Autodesk Fusion 360 part; units mm, degrees
(part 11 of 18)
  line L7284 (210.9744, -11.8381) -> (210.7744, -11.8381)
  line L7285 (210.7744, -11.8381) -> (210.7744, -12.5031)
  line L7286 (211.1744, -11.8381) -> (211.1744, -12.5031)
  line L7287 (211.1744, -12.5031) -> (211.3744, -12.5031)
  line L7288 (211.3744, -12.5031) -> (211.3744, -11.8381)
  line L7289 (211.3744, -11.8381) -> (211.1744, -11.8381)
  line L7290 (208.5746, -11.8381) -> (208.3746, -11.8381)
  line L7291 (208.3746, -11.8381) -> (208.3746, -12.5031)
  line L7292 (208.5746, -12.5031) -> (208.5746, -11.8381)
  line L7293 (208.3746, -12.5031) -> (208.5746, -12.5031)
  line L7294 (213.3744, -11.8381) -> (213.1744, -11.8381)
  line L7295 (213.1744, -11.8381) -> (213.1744, -12.5031)
  line L7296 (213.3744, -12.5031) -> (213.3744, -11.8381)
  line L7297 (213.1744, -12.5031) -> (213.3744, -12.5031)
  line L7298 (210.3746, -12.5031) -> (210.5746, -12.5031)
  line L7299 (210.5746, -11.8381) -> (210.3746, -11.8381)
  line L7300 (210.5746, -12.5031) -> (210.5746, -11.8381)
  line L7301 (210.3746, -11.8381) -> (210.3746, -12.5031)
  line L7302 (212.9744, -11.8381) -> (212.7744, -11.8381)
  line L7303 (212.7744, -11.8381) -> (212.7744, -12.5031)
  line L7304 (212.7744, -12.5031) -> (212.9744, -12.5031)
  line L7305 (212.9744, -12.5031) -> (212.9744, -11.8381)
  line L7306 (210.1745, -12.5031) -> (210.1745, -11.8381)
  line L7307 (209.9745, -12.5031) -> (210.1745, -12.5031)
  line L7308 (210.1745, -11.8381) -> (209.9745, -11.8381)
  line L7309 (209.9745, -11.8381) -> (209.9745, -12.5031)
  line L7310 (212.5746, -11.8381) -> (212.3746, -11.8381)
  line L7311 (212.3746, -12.5031) -> (212.5746, -12.5031)
  line L7312 (212.3746, -11.8381) -> (212.3746, -12.5031)
  line L7313 (212.5746, -12.5031) -> (212.5746, -11.8381)
  line L7314 (209.5745, -11.8381) -> (209.5745, -12.5031)
  line L7315 (209.7745, -12.5031) -> (209.7745, -11.8381)
  line L7316 (209.5745, -12.5031) -> (209.7745, -12.5031)
  line L7317 (209.7745, -11.8381) -> (209.5745, -11.8381)
  line L7318 (211.5745, -11.8381) -> (211.5745, -12.5031)
  line L7319 (211.5745, -12.5031) -> (211.7745, -12.5031)
  line L7320 (211.7745, -11.8381) -> (211.5745, -11.8381)
  line L7321 (211.7745, -12.5031) -> (211.7745, -11.8381)
  line L7322 (208.9744, -12.5031) -> (208.9744, -11.8381)
  line L7323 (208.9744, -11.8381) -> (208.7744, -11.8381)
  line L7324 (208.7744, -11.8381) -> (208.7744, -12.5031)
  line L7325 (208.7744, -12.5031) -> (208.9744, -12.5031)
  line L7326 (211.9745, -11.8381) -> (211.9745, -12.5031)
  line L7327 (212.1745, -12.5031) -> (212.1745, -11.8381)
  line L7328 (212.1745, -11.8381) -> (211.9745, -11.8381)
  line L7329 (211.9745, -12.5031) -> (212.1745, -12.5031)
  line L7330 (209.3744, -12.5031) -> (209.3744, -11.8381)
  line L7331 (209.1744, -12.5031) -> (209.3744, -12.5031)
  line L7332 (209.1744, -11.8381) -> (209.1744, -12.5031)
  line L7333 (209.3744, -11.8381) -> (209.1744, -11.8381)
  line L7334 (209.4745, -7.1629) -> (212.6745, -7.1629)
  line L7335 (212.6745, -7.1629) -> (212.6745, -10.3629)
  line L7336 (212.6745, -10.3629) -> (209.4745, -10.3629)
  line L7337 (209.4745, -10.3629) -> (209.4745, -7.1629)
  line L7338 (188.0514, -6.559) -> (188.4214, -6.559)
  line L7339 (188.0514, -7.131) -> (188.1014, -7.181)
  line L7340 (188.4214, -6.889) -> (188.0514, -6.889)
  line L7341 (188.1014, -7.181) -> (188.9014, -7.181)
  line L7342 (188.4214, -6.559) -> (188.4214, -6.889)
  line L7343 (188.9514, -6.331) -> (188.9014, -6.281)
  line L7344 (188.9014, -7.181) -> (188.9514, -7.131)
  line L7345 (188.9014, -6.281) -> (188.1014, -6.281)
  line L7346 (188.0514, -6.889) -> (188.0514, -7.131)
  line L7347 (188.9514, -7.131) -> (188.9514, -6.331)
  line L7348 (188.1014, -6.281) -> (188.0514, -6.331)
  line L7349 (188.0514, -6.331) -> (188.0514, -6.559)
  line L7350 (187.3114, -7.181) -> (187.3614, -7.131)
  line L7351 (186.4614, -7.131) -> (186.5114, -7.181)
  line L7352 (186.5114, -6.281) -> (186.4614, -6.331)
  line L7353 (186.9914, -6.903) -> (186.9914, -6.573)
  line L7354 (186.5114, -7.181) -> (187.3114, -7.181)
  line L7355 (187.3614, -6.331) -> (187.3114, -6.281)
  line L7356 (187.3114, -6.281) -> (186.5114, -6.281)
  line L7357 (187.3614, -7.131) -> (187.3614, -6.903)
  line L7358 (186.4614, -6.331) -> (186.4614, -7.131)
  line L7359 (186.9914, -6.573) -> (187.3614, -6.573)
  line L7360 (187.3614, -6.903) -> (186.9914, -6.903)
  line L7361 (187.3614, -6.573) -> (187.3614, -6.331)
  line L7362 (181.9393, -7.181) -> (182.7393, -7.181)
  line L7363 (181.9393, -6.281) -> (181.8894, -6.331)
  line L7364 (182.4194, -6.573) -> (182.7894, -6.573)
  line L7365 (181.8894, -6.331) -> (181.8894, -7.131)
  line L7366 (182.7894, -6.331) -> (182.7393, -6.281)
  line L7367 (182.7894, -6.903) -> (182.4194, -6.903)
  line L7368 (182.7894, -7.131) -> (182.7894, -6.903)
  line L7369 (182.7393, -6.281) -> (181.9393, -6.281)
  line L7370 (182.4194, -6.903) -> (182.4194, -6.573)
  line L7371 (182.7393, -7.181) -> (182.7894, -7.131)
  line L7372 (182.7894, -6.573) -> (182.7894, -6.331)
  line L7373 (181.8894, -7.131) -> (181.9393, -7.181)
  line L7374 (183.8494, -6.559) -> (183.8494, -6.889)
  line L7375 (183.4794, -6.559) -> (183.8494, -6.559)
  line L7376 (183.4794, -6.331) -> (183.4794, -6.559)
  line L7377 (184.3294, -6.281) -> (183.5294, -6.281)
  line L7378 (183.4794, -6.889) -> (183.4794, -7.131)
  line L7379 (183.4794, -7.131) -> (183.5294, -7.181)
  line L7380 (183.5294, -7.181) -> (184.3294, -7.181)
  line L7381 (184.3294, -7.181) -> (184.3794, -7.131)
  line L7382 (183.8494, -6.889) -> (183.4794, -6.889)
  line L7383 (183.5294, -6.281) -> (183.4794, -6.331)
  line L7384 (184.3794, -6.331) -> (184.3294, -6.281)
  line L7385 (184.3794, -7.131) -> (184.3794, -6.331)
  line L7386 (-10.6934, -88.5446) -> (-10.6934, 1.6256)
  line L7387 (222.987, 1.6256) -> (222.987, -88.5446)
  line L7388 (-10.6934, 1.6256) -> (222.987, 1.6256)
  line L7389 (222.987, -88.5446) -> (-10.6934, -88.5446)
  arc A1072 (188.2393, -3.84) -> (188.8893, -3.84) centre (188.5643, -3.84) ccw
  arc A1073 (188.8893, -3.84) -> (188.2393, -3.84) centre (188.5643, -3.84) ccw
  arc A1074 (182.4592, -3.84) -> (183.1092, -3.84) centre (182.7842, -3.84) ccw
  arc A1075 (183.1092, -3.84) -> (182.4592, -3.84) centre (182.7842, -3.84) ccw
  arc A1076 (194.3974, -57.5184) -> (189.3974, -57.5184) centre (191.8974, -57.5184) ccw
  arc A1077 (189.3974, -57.5184) -> (194.3974, -57.5184) centre (191.8974, -57.5184) ccw
  arc A1078 (170.3473, -76.5812) -> (175.3474, -76.5812) centre (172.8473, -76.5812) ccw
  arc A1079 (175.3474, -76.5812) -> (170.3473, -76.5812) centre (172.8473, -76.5812) ccw
  arc A1080 (175.3474, -57.5184) -> (170.3473, -57.5184) centre (172.8473, -57.5184) ccw
  arc A1081 (170.3473, -57.5184) -> (175.3474, -57.5184) centre (172.8473, -57.5184) ccw
  arc A1082 (175.3474, -38.4557) -> (170.3473, -38.4557) centre (172.8473, -38.4557) ccw
  arc A1083 (170.3473, -38.4557) -> (175.3474, -38.4557) centre (172.8473, -38.4557) ccw
  arc A1084 (170.3473, -19.4056) -> (175.3474, -19.4056) centre (172.8473, -19.4056) ccw
  arc A1085 (175.3474, -19.4056) -> (170.3473, -19.4056) centre (172.8473, -19.4056) ccw
  arc A1086 (151.2973, -76.5812) -> (156.2973, -76.5812) centre (153.7973, -76.5812) ccw
  arc A1087 (156.2973, -76.5812) -> (151.2973, -76.5812) centre (153.7973, -76.5812) ccw
  arc A1088 (156.2973, -38.4557) -> (151.2973, -38.4557) centre (153.7973, -38.4557) ccw
  arc A1089 (151.2973, -38.4557) -> (156.2973, -38.4557) centre (153.7973, -38.4557) ccw
  arc A1090 (156.2973, -57.5184) -> (151.2973, -57.5184) centre (153.7973, -57.5184) ccw
  arc A1091 (151.2973, -57.5184) -> (156.2973, -57.5184) centre (153.7973, -57.5184) ccw
  arc A1092 (156.2973, -19.4056) -> (151.2973, -19.4056) centre (153.7973, -19.4056) ccw
  arc A1093 (151.2973, -19.4056) -> (156.2973, -19.4056) centre (153.7973, -19.4056) ccw
  arc A1094 (132.2473, -57.5184) -> (137.2473, -57.5184) centre (134.7473, -57.5184) ccw
  arc A1095 (137.2473, -57.5184) -> (132.2473, -57.5184) centre (134.7473, -57.5184) ccw
  arc A1096 (137.2473, -38.4557) -> (132.2473, -38.4557) centre (134.7473, -38.4557) ccw
  arc A1097 (132.2473, -38.4557) -> (137.2473, -38.4557) centre (134.7473, -38.4557) ccw
  arc A1098 (132.2473, -19.4056) -> (137.2473, -19.4056) centre (134.7473, -19.4056) ccw
  arc A1099 (137.2473, -19.4056) -> (132.2473, -19.4056) centre (134.7473, -19.4056) ccw
  arc A1100 (132.2473, -76.5812) -> (137.2473, -76.5812) centre (134.7473, -76.5812) ccw
  arc A1101 (137.2473, -76.5812) -> (132.2473, -76.5812) centre (134.7473, -76.5812) ccw
  arc A1102 (118.1972, -76.5812) -> (113.1972, -76.5812) centre (115.6972, -76.5812) ccw
  arc A1103 (113.1972, -76.5812) -> (118.1972, -76.5812) centre (115.6972, -76.5812) ccw
  line L7390 (118.1972, -76.5812) -> (118.1972, -76.5812)
  arc A1104 (118.1972, -57.5184) -> (113.1972, -57.5184) centre (115.6972, -57.5184) ccw
  line L7391 (118.1972, -57.5184) -> (118.1972, -57.5184)
  arc A1105 (113.1972, -57.5184) -> (118.1972, -57.5184) centre (115.6972, -57.5184) ccw
  arc A1106 (113.1972, -19.4056) -> (118.1972, -19.4056) centre (115.6972, -19.4056) ccw
  arc A1107 (118.1972, -19.4056) -> (113.1972, -19.4056) centre (115.6972, -19.4056) ccw
  line L7392 (118.1972, -19.4056) -> (118.1972, -19.4056)
  line L7393 (118.1972, -38.4557) -> (118.1972, -38.4557)
  arc A1108 (113.1972, -38.4557) -> (118.1972, -38.4557) centre (115.6972, -38.4557) ccw
  arc A1109 (118.1972, -38.4557) -> (113.1972, -38.4557) centre (115.6972, -38.4557) ccw
  arc A1110 (94.1472, -19.4056) -> (99.1472, -19.4056) centre (96.6472, -19.4056) ccw
  arc A1111 (99.1472, -19.4056) -> (94.1472, -19.4056) centre (96.6472, -19.4056) ccw
  line L7394 (99.1472, -19.4056) -> (99.1472, -19.4056)
  line L7395 (99.1472, -38.4557) -> (99.1472, -38.4557)
  arc A1112 (94.1472, -38.4557) -> (99.1472, -38.4557) centre (96.6472, -38.4557) ccw
  arc A1113 (99.1472, -38.4557) -> (94.1472, -38.4557) centre (96.6472, -38.4557) ccw
  line L7396 (99.1472, -76.5812) -> (99.1472, -76.5812)
  arc A1114 (99.1472, -76.5812) -> (94.1472, -76.5812) centre (96.6472, -76.5812) ccw
  arc A1115 (94.1472, -76.5812) -> (99.1472, -76.5812) centre (96.6472, -76.5812) ccw
  line L7397 (99.1472, -57.5184) -> (99.1472, -57.5184)
  arc A1116 (99.1472, -57.5184) -> (94.1472, -57.5184) centre (96.6472, -57.5184) ccw
  arc A1117 (94.1472, -57.5184) -> (99.1472, -57.5184) centre (96.6472, -57.5184) ccw
  arc A1118 (194.3974, -76.5812) -> (189.3974, -76.5812) centre (191.8974, -76.5812) ccw
  arc A1119 (189.3974, -76.5812) -> (194.3974, -76.5812) centre (191.8974, -76.5812) ccw
  arc A1120 (189.3974, -19.4056) -> (194.3974, -19.4056) centre (191.8974, -19.4056) ccw
  arc A1121 (194.3974, -19.4056) -> (189.3974, -19.4056) centre (191.8974, -19.4056) ccw
  line L7398 (80.0972, -76.5812) -> (80.0972, -76.5812)
  arc A1122 (75.0972, -76.5812) -> (80.0972, -76.5812) centre (77.5972, -76.5812) ccw
  arc A1123 (80.0972, -76.5812) -> (75.0972, -76.5812) centre (77.5972, -76.5812) ccw
  arc A1124 (80.0972, -38.4557) -> (75.0972, -38.4557) centre (77.5972, -38.4557) ccw
  line L7399 (80.0972, -38.4557) -> (80.0972, -38.4557)
  arc A1125 (75.0972, -38.4557) -> (80.0972, -38.4557) centre (77.5972, -38.4557) ccw
  arc A1126 (75.0972, -19.4056) -> (80.0972, -19.4056) centre (77.5972, -19.4056) ccw
  line L7400 (80.0972, -19.4056) -> (80.0972, -19.4056)
  arc A1127 (80.0972, -19.4056) -> (75.0972, -19.4056) centre (77.5972, -19.4056) ccw
  arc A1128 (80.0972, -57.5184) -> (75.0972, -57.5184) centre (77.5972, -57.5184) ccw
  arc A1129 (75.0972, -57.5184) -> (80.0972, -57.5184) centre (77.5972, -57.5184) ccw
  line L7401 (80.0972, -57.5184) -> (80.0972, -57.5184)
  arc A1130 (56.0471, -76.5812) -> (61.0471, -76.5812) centre (58.5471, -76.5812) ccw
  arc A1131 (61.0471, -76.5812) -> (56.0471, -76.5812) centre (58.5471, -76.5812) ccw
  arc A1132 (61.0471, -57.5184) -> (56.0471, -57.5184) centre (58.5471, -57.5184) ccw
  arc A1133 (56.0471, -57.5184) -> (61.0471, -57.5184) centre (58.5471, -57.5184) ccw
  arc A1134 (61.0471, -38.4557) -> (56.0471, -38.4557) centre (58.5471, -38.4557) ccw
  arc A1135 (56.0471, -38.4557) -> (61.0471, -38.4557) centre (58.5471, -38.4557) ccw
  arc A1136 (41.9971, -57.5184) -> (36.9971, -57.5184) centre (39.4971, -57.5184) ccw
  arc A1137 (36.9971, -57.5184) -> (41.9971, -57.5184) centre (39.4971, -57.5184) ccw
  arc A1138 (36.9971, -76.5812) -> (41.9971, -76.5812) centre (39.4971, -76.5812) ccw
  arc A1139 (41.9971, -76.5812) -> (36.9971, -76.5812) centre (39.4971, -76.5812) ccw
  arc A1140 (22.947, -76.5812) -> (17.947, -76.5812) centre (20.447, -76.5812) ccw
  arc A1141 (17.947, -76.5812) -> (22.947, -76.5812) centre (20.447, -76.5812) ccw
  arc A1142 (3.897, -76.5812) -> (-1.103, -76.5812) centre (1.397, -76.5812) ccw
  arc A1143 (-1.103, -76.5812) -> (3.897, -76.5812) centre (1.397, -76.5812) ccw
  arc A1144 (61.0471, -19.4056) -> (56.0471, -19.4056) centre (58.5471, -19.4056) ccw
  arc A1145 (56.0471, -19.4056) -> (61.0471, -19.4056) centre (58.5471, -19.4056) ccw
  arc A1146 (36.9971, -38.4557) -> (41.9971, -38.4557) centre (39.4971, -38.4557) ccw
  arc A1147 (41.9971, -38.4557) -> (36.9971, -38.4557) centre (39.4971, -38.4557) ccw
  arc A1148 (36.9971, -19.4056) -> (41.9971, -19.4056) centre (39.4971, -19.4056) ccw
  arc A1149 (41.9971, -19.4056) -> (36.9971, -19.4056) centre (39.4971, -19.4056) ccw
  arc A1150 (22.947, -19.4056) -> (17.947, -19.4056) centre (20.447, -19.4056) ccw
  arc A1151 (17.947, -19.4056) -> (22.947, -19.4056) centre (20.447, -19.4056) ccw
  arc A1152 (22.947, -57.5184) -> (17.947, -57.5184) centre (20.447, -57.5184) ccw
  arc A1153 (17.947, -57.5184) -> (22.947, -57.5184) centre (20.447, -57.5184) ccw
  arc A1154 (17.947, -38.4557) -> (22.947, -38.4557) centre (20.447, -38.4557) ccw
  arc A1155 (22.947, -38.4557) -> (17.947, -38.4557) centre (20.447, -38.4557) ccw
  arc A1156 (3.897, -19.4056) -> (-1.103, -19.4056) centre (1.397, -19.4056) ccw
  arc A1157 (-1.103, -19.4056) -> (3.897, -19.4056) centre (1.397, -19.4056) ccw
  arc A1158 (-1.103, -38.4557) -> (3.897, -38.4557) centre (1.397, -38.4557) ccw
  arc A1159 (3.897, -38.4557) -> (-1.103, -38.4557) centre (1.397, -38.4557) ccw
  arc A1160 (3.897, -57.5184) -> (-1.103, -57.5184) centre (1.397, -57.5184) ccw
  arc A1161 (-1.103, -57.5184) -> (3.897, -57.5184) centre (1.397, -57.5184) ccw
  arc A1162 (208.4474, -57.5184) -> (213.4474, -57.5184) centre (210.9474, -57.5184) ccw
  arc A1163 (213.4474, -57.5184) -> (208.4474, -57.5184) centre (210.9474, -57.5184) ccw
  arc A1164 (213.4474, -38.4557) -> (208.4474, -38.4557) centre (210.9474, -38.4557) ccw
  arc A1165 (208.4474, -38.4557) -> (213.4474, -38.4557) centre (210.9474, -38.4557) ccw
  arc A1166 (213.4474, -19.4056) -> (208.4474, -19.4056) centre (210.9474, -19.4056) ccw
  arc A1167 (208.4474, -19.4056) -> (213.4474, -19.4056) centre (210.9474, -19.4056) ccw
  arc A1168 (213.4474, -76.5812) -> (208.4474, -76.5812) centre (210.9474, -76.5812) ccw
  arc A1169 (208.4474, -76.5812) -> (213.4474, -76.5812) centre (210.9474, -76.5812) ccw
  arc A1170 (194.3974, -38.4557) -> (189.3974, -38.4557) centre (191.8974, -38.4557) ccw
  arc A1171 (189.3974, -38.4557) -> (194.3974, -38.4557) centre (191.8974, -38.4557) ccw
  line L7402 (189.518, -5.1651) -> (189.4443, -4.8901)
  line L7403 (190.4706, -5.1651) -> (190.2693, -5.3664)
  line L7404 (189.4443, -3.7901) -> (189.518, -3.5151)
  line L7405 (190.4706, -3.5151) -> (190.5443, -3.7901)
  line L7406 (189.7193, -5.3664) -> (189.518, -5.1651)
  line L7407 (189.518, -3.5151) -> (189.7193, -3.3138)
  line L7408 (189.4443, -4.8901) -> (189.4443, -3.7901)
  line L7409 (190.2693, -5.3664) -> (189.9943, -5.4401)
  line L7410 (190.5443, -3.7901) -> (190.5443, -4.8901)
  line L7411 (190.5443, -4.8901) -> (190.4706, -5.1651)
  line L7412 (190.2693, -3.3138) -> (190.4706, -3.5151)
  line L7413 (189.9943, -5.4401) -> (189.7193, -5.3664)
  line L7414 (189.9943, -3.2401) -> (190.2693, -3.3138)
  line L7415 (189.7193, -3.3138) -> (189.9943, -3.2401)
  line L7416 (190.5443, -3.7901) -> (190.5443, -4.8901)
  line L7417 (189.4443, -4.8901) -> (189.4443, -3.7901)
  line L7418 (189.518, -5.1651) -> (189.4443, -4.8901)
  line L7419 (189.7193, -3.3138) -> (189.9943, -3.2401)
  line L7420 (189.518, -3.5151) -> (189.7193, -3.3138)
  line L7421 (189.9943, -3.2401) -> (190.2693, -3.3138)
  line L7422 (190.4706, -3.5151) -> (190.5443, -3.7901)
  line L7423 (189.9943, -5.4401) -> (189.7193, -5.3664)
  line L7424 (190.2693, -3.3138) -> (190.4706, -3.5151)
  line L7425 (189.4443, -3.7901) -> (189.518, -3.5151)
  line L7426 (189.7193, -5.3664) -> (189.518, -5.1651)
  line L7427 (190.4706, -5.1651) -> (190.2693, -5.3664)
  line L7428 (190.5443, -4.8901) -> (190.4706, -5.1651)
  line L7429 (190.2693, -5.3664) -> (189.9943, -5.4401)
  line L7430 (190.2693, -5.3664) -> (189.9943, -5.4401)
  line L7431 (189.518, -5.1651) -> (189.4443, -4.8901)
  line L7432 (190.2693, -3.3138) -> (190.4706, -3.5151)
  line L7433 (189.7193, -5.3664) -> (189.518, -5.1651)
  line L7434 (189.4443, -3.7901) -> (189.518, -3.5151)
  line L7435 (189.7193, -3.3138) -> (189.9943, -3.2401)
  line L7436 (190.4706, -5.1651) -> (190.2693, -5.3664)
  line L7437 (189.9943, -3.2401) -> (190.2693, -3.3138)
  line L7438 (189.9943, -5.4401) -> (189.7193, -5.3664)
  line L7439 (190.4706, -3.5151) -> (190.5443, -3.7901)
  line L7440 (189.518, -3.5151) -> (189.7193, -3.3138)
  line L7441 (190.5443, -3.7901) -> (190.5443, -4.8901)
  line L7442 (190.5443, -4.8901) -> (190.4706, -5.1651)
  line L7443 (189.4443, -4.8901) -> (189.4443, -3.7901)
  line L7444 (180.8045, -4.8901) -> (180.8045, -3.7901)
  line L7445 (181.9045, -4.8901) -> (181.8308, -5.1651)
  line L7446 (181.0795, -3.3138) -> (181.3545, -3.2401)
  line L7447 (181.6295, -5.3664) -> (181.3545, -5.4401)
  line L7448 (181.3545, -5.4401) -> (181.0795, -5.3664)
  line L7449 (181.3545, -3.2401) -> (181.6295, -3.3138)
  line L7450 (181.6295, -3.3138) -> (181.8308, -3.5151)
  line L7451 (181.8308, -3.5151) -> (181.9045, -3.7901)
  line L7452 (181.9045, -3.7901) -> (181.9045, -4.8901)
  line L7453 (181.0795, -5.3664) -> (180.8781, -5.1651)
  line L7454 (181.8308, -5.1651) -> (181.6295, -5.3664)
  line L7455 (180.8781, -5.1651) -> (180.8045, -4.8901)
  line L7456 (180.8781, -3.5151) -> (181.0795, -3.3138)
  line L7457 (180.8045, -3.7901) -> (180.8781, -3.5151)
  line L7458 (181.8308, -3.5151) -> (181.9045, -3.7901)
  line L7459 (181.3545, -5.4401) -> (181.0795, -5.3664)
  line L7460 (180.8781, -5.1651) -> (180.8045, -4.8901)
  line L7461 (180.8781, -3.5151) -> (181.0795, -3.3138)
  line L7462 (181.3545, -3.2401) -> (181.6295, -3.3138)
  line L7463 (181.9045, -3.7901) -> (181.9045, -4.8901)
  line L7464 (181.0795, -3.3138) -> (181.3545, -3.2401)
  line L7465 (181.9045, -4.8901) -> (181.8308, -5.1651)
  line L7466 (180.8045, -4.8901) -> (180.8045, -3.7901)
  line L7467 (181.6295, -3.3138) -> (181.8308, -3.5151)
  line L7468 (181.8308, -5.1651) -> (181.6295, -5.3664)
  line L7469 (181.6295, -5.3664) -> (181.3545, -5.4401)
  line L7470 (180.8045, -3.7901) -> (180.8781, -3.5151)
  line L7471 (181.0795, -5.3664) -> (180.8781, -5.1651)
  line L7472 (181.0795, -5.3664) -> (180.8781, -5.1651)
  line L7473 (181.9045, -4.8901) -> (181.8308, -5.1651)
  line L7474 (181.6295, -5.3664) -> (181.3545, -5.4401)
  line L7475 (180.8781, -5.1651) -> (180.8045, -4.8901)
  line L7476 (181.3545, -5.4401) -> (181.0795, -5.3664)
  line L7477 (181.8308, -3.5151) -> (181.9045, -3.7901)
  line L7478 (180.8045, -4.8901) -> (180.8045, -3.7901)
  line L7479 (180.8781, -3.5151) -> (181.0795, -3.3138)
  line L7480 (180.8045, -3.7901) -> (180.8781, -3.5151)
  line L7481 (181.3545, -3.2401) -> (181.6295, -3.3138)
  line L7482 (181.9045, -3.7901) -> (181.9045, -4.8901)
  line L7483 (181.6295, -3.3138) -> (181.8308, -3.5151)
  line L7484 (181.0795, -3.3138) -> (181.3545, -3.2401)
  line L7485 (181.8308, -5.1651) -> (181.6295, -5.3664)
  line L7486 (189.9943, 0.76) -> (190.2693, 0.6863)
  line L7487 (189.518, 0.485) -> (189.7193, 0.6863)
  line L7488 (189.518, -0.865) -> (189.4443, -0.59)
  line L7489 (190.5443, 0.21) -> (190.5443, -0.59)
  line L7490 (190.4706, 0.485) -> (190.5443, 0.21)
  line L7491 (190.4706, -0.865) -> (190.2693, -1.0663)
  line L7492 (190.2693, -1.0663) -> (189.9943, -1.14)
  line L7493 (189.4443, 0.21) -> (189.518, 0.485)
  line L7494 (189.7193, 0.6863) -> (189.9943, 0.76)
  line L7495 (190.5443, -0.59) -> (190.4706, -0.865)
  line L7496 (189.7193, -1.0663) -> (189.518, -0.865)
  line L7497 (189.9943, -1.14) -> (189.7193, -1.0663)
  line L7498 (189.4443, -0.59) -> (189.4443, 0.21)
  line L7499 (190.2693, 0.6863) -> (190.4706, 0.485)
  line L7500 (190.4706, 0.485) -> (190.5443, 0.21)
  line L7501 (189.7193, -1.0663) -> (189.518, -0.865)
  line L7502 (189.4443, -0.59) -> (189.4443, 0.21)
  line L7503 (189.4443, 0.21) -> (189.518, 0.485)
  line L7504 (189.9943, -1.14) -> (189.7193, -1.0663)
  line L7505 (189.7193, 0.6863) -> (189.9943, 0.76)
  line L7506 (189.9943, 0.76) -> (190.2693, 0.6863)
  line L7507 (190.5443, 0.21) -> (190.5443, -0.59)
  line L7508 (189.518, -0.865) -> (189.4443, -0.59)
  line L7509 (190.2693, 0.6863) -> (190.4706, 0.485)
  line L7510 (190.4706, -0.865) -> (190.2693, -1.0663)
  line L7511 (190.2693, -1.0663) -> (189.9943, -1.14)
  line L7512 (190.5443, -0.59) -> (190.4706, -0.865)
  line L7513 (189.518, 0.485) -> (189.7193, 0.6863)
  line L7514 (190.5443, -0.59) -> (190.4706, -0.865)
  line L7515 (189.518, -0.865) -> (189.4443, -0.59)
  line L7516 (189.4443, -0.59) -> (189.4443, 0.21)
  line L7517 (190.5443, 0.21) -> (190.5443, -0.59)
  line L7518 (189.7193, -1.0663) -> (189.518, -0.865)
  line L7519 (190.2693, -1.0663) -> (189.9943, -1.14)
  line L7520 (189.7193, 0.6863) -> (189.9943, 0.76)
  line L7521 (189.9943, 0.76) -> (190.2693, 0.6863)
  line L7522 (190.2693, 0.6863) -> (190.4706, 0.485)
  line L7523 (189.4443, 0.21) -> (189.518, 0.485)
  line L7524 (189.518, 0.485) -> (189.7193, 0.6863)
  line L7525 (190.4706, -0.865) -> (190.2693, -1.0663)
  line L7526 (189.9943, -1.14) -> (189.7193, -1.0663)
  line L7527 (190.4706, 0.485) -> (190.5443, 0.21)
  line L7528 (180.8045, 0.21) -> (180.8781, 0.485)
  line L7529 (181.8308, -0.865) -> (181.6295, -1.0663)
  line L7530 (181.3545, -1.14) -> (181.0795, -1.0663)
  line L7531 (181.0795, -1.0663) -> (180.8781, -0.865)
  line L7532 (180.8781, 0.485) -> (181.0795, 0.6863)
  line L7533 (181.3545, 0.76) -> (181.6295, 0.6863)
  line L7534 (181.6295, 0.6863) -> (181.8308, 0.485)
  line L7535 (181.0795, 0.6863) -> (181.3545, 0.76)
  line L7536 (181.9045, 0.21) -> (181.9045, -0.59)
  line L7537 (181.6295, -1.0663) -> (181.3545, -1.14)
  line L7538 (180.8045, -0.59) -> (180.8045, 0.21)
  line L7539 (181.9045, -0.59) -> (181.8308, -0.865)
  line L7540 (181.8308, 0.485) -> (181.9045, 0.21)
  line L7541 (180.8781, -0.865) -> (180.8045, -0.59)
  line L7542 (180.8781, 0.485) -> (181.0795, 0.6863)
  line L7543 (181.6295, 0.6863) -> (181.8308, 0.485)
  line L7544 (180.8045, 0.21) -> (180.8781, 0.485)
  line L7545 (181.6295, -1.0663) -> (181.3545, -1.14)
  line L7546 (181.8308, 0.485) -> (181.9045, 0.21)
  line L7547 (181.3545, -1.14) -> (181.0795, -1.0663)
  line L7548 (181.0795, 0.6863) -> (181.3545, 0.76)
  line L7549 (181.9045, 0.21) -> (181.9045, -0.59)
  line L7550 (180.8045, -0.59) -> (180.8045, 0.21)
  line L7551 (181.8308, -0.865) -> (181.6295, -1.0663)
  line L7552 (180.8781, -0.865) -> (180.8045, -0.59)
  line L7553 (181.9045, -0.59) -> (181.8308, -0.865)
  line L7554 (181.0795, -1.0663) -> (180.8781, -0.865)
  line L7555 (181.3545, 0.76) -> (181.6295, 0.6863)
  line L7556 (180.8781, 0.485) -> (181.0795, 0.6863)
  line L7557 (181.8308, 0.485) -> (181.9045, 0.21)
  line L7558 (181.9045, 0.21) -> (181.9045, -0.59)
  line L7559 (181.9045, -0.59) -> (181.8308, -0.865)
  line L7560 (181.3545, 0.76) -> (181.6295, 0.6863)
  line L7561 (181.6295, 0.6863) -> (181.8308, 0.485)
  line L7562 (181.3545, -1.14) -> (181.0795, -1.0663)
  line L7563 (181.6295, -1.0663) -> (181.3545, -1.14)
  line L7564 (181.8308, -0.865) -> (181.6295, -1.0663)
  line L7565 (180.8781, -0.865) -> (180.8045, -0.59)
  line L7566 (181.0795, -1.0663) -> (180.8781, -0.865)
  line L7567 (180.8045, 0.21) -> (180.8781, 0.485)
  line L7568 (181.0795, 0.6863) -> (181.3545, 0.76)
  line L7569 (180.8045, -0.59) -> (180.8045, 0.21)
  arc A1172 (10.5631, -8.0011) -> (8.7631, -8.0011) centre (9.6631, -8.0011) ccw
  arc A1173 (8.7631, -8.0011) -> (10.5631, -8.0011) centre (9.6631, -8.0011) ccw
  arc A1174 (10.5631, -8.0011) -> (8.7631, -8.0011) centre (9.6631, -8.0011) ccw
  arc A1175 (8.7631, -8.0011) -> (10.5631, -8.0011) centre (9.6631, -8.0011) ccw
  arc A1176 (10.5631, -8.0011) -> (8.7631, -8.0011) centre (9.6631, -8.0011) ccw
  arc A1177 (8.7631, -8.0011) -> (10.5631, -8.0011) centre (9.6631, -8.0011) ccw
  arc A1178 (10.5631, -5.4611) -> (8.7631, -5.4611) centre (9.6631, -5.4611) ccw
  arc A1179 (8.7631, -5.4611) -> (10.5631, -5.4611) centre (9.6631, -5.4611) ccw
  arc A1180 (10.5631, -5.4611) -> (8.7631, -5.4611) centre (9.6631, -5.4611) ccw
  arc A1181 (8.7631, -5.4611) -> (10.5631, -5.4611) centre (9.6631, -5.4611) ccw
  arc A1182 (8.7631, -5.4611) -> (10.5631, -5.4611) centre (9.6631, -5.4611) ccw
  arc A1183 (10.5631, -5.4611) -> (8.7631, -5.4611) centre (9.6631, -5.4611) ccw
  arc A1184 (10.5631, -2.9211) -> (8.7631, -2.9211) centre (9.6631, -2.9211) ccw
  arc A1185 (8.7631, -2.9211) -> (10.5631, -2.9211) centre (9.6631, -2.9211) ccw
  arc A1186 (10.5631, -2.9211) -> (8.7631, -2.9211) centre (9.6631, -2.9211) ccw
  arc A1187 (8.7631, -2.9211) -> (10.5631, -2.9211) centre (9.6631, -2.9211) ccw
  arc A1188 (8.7631, -2.9211) -> (10.5631, -2.9211) centre (9.6631, -2.9211) ccw
  arc A1189 (10.5631, -2.9211) -> (8.7631, -2.9211) centre (9.6631, -2.9211) ccw
  line L7570 (-3.9371, -8.0011) -> (-3.9371, -8.0011)
  arc A1190 (-3.9371, -8.0011) -> (-5.7371, -8.0011) centre (-4.8371, -8.0011) ccw
  arc A1191 (-5.7371, -8.0011) -> (-3.9371, -8.0011) centre (-4.8371, -8.0011) ccw
  arc A1192 (-5.7371, -8.0011) -> (-3.9371, -8.0011) centre (-4.8371, -8.0011) ccw
  line L7571 (-3.9371, -8.0011) -> (-3.9371, -8.0011)
  arc A1193 (-3.9371, -8.0011) -> (-5.7371, -8.0011) centre (-4.8371, -8.0011) ccw
  arc A1194 (-3.9371, -8.0011) -> (-5.7371, -8.0011) centre (-4.8371, -8.0011) ccw
  line L7572 (-3.9371, -8.0011) -> (-3.9371, -8.0011)
  arc A1195 (-5.7371, -8.0011) -> (-3.9371, -8.0011) centre (-4.8371, -8.0011) ccw
  arc A1196 (-3.9371, -2.9211) -> (-5.7371, -2.9211) centre (-4.8371, -2.9211) ccw
  line L7573 (-3.9371, -2.9211) -> (-3.9371, -2.9211)
  arc A1197 (-5.7371, -2.9211) -> (-3.9371, -2.9211) centre (-4.8371, -2.9211) ccw
  line L7574 (-3.9371, -2.9211) -> (-3.9371, -2.9211)
  arc A1198 (-3.9371, -2.9211) -> (-5.7371, -2.9211) centre (-4.8371, -2.9211) ccw
  arc A1199 (-5.7371, -2.9211) -> (-3.9371, -2.9211) centre (-4.8371, -2.9211) ccw
  arc A1200 (-3.9371, -2.9211) -> (-5.7371, -2.9211) centre (-4.8371, -2.9211) ccw
  line L7575 (-3.9371, -2.9211) -> (-3.9371, -2.9211)
  arc A1201 (-5.7371, -2.9211) -> (-3.9371, -2.9211) centre (-4.8371, -2.9211) ccw
  line L7576 (4.0754, -0.4011) -> (3.8261, -0.7742)
  line L7577 (0.1629, 0.039) -> (0.2505, 0.4791)
  line L7578 (0.8729, 1.1015) -> (1.3129, 1.189)
  line L7579 (4.0754, 0.4791) -> (4.1629, 0.039)
  line L7580 (3.8261, 0.8522) -> (4.0754, 0.4791)
  line L7581 (0.4998, 0.8522) -> (0.8729, 1.1015)
  line L7582 (0.4998, -0.7742) -> (0.2505, -0.4011)
  line L7583 (0.8729, -1.0235) -> (0.4998, -0.7742)
  line L7584 (4.1629, 0.039) -> (4.0754, -0.4011)
  line L7585 (3.453, -1.0235) -> (3.0129, -1.111)
  line L7586 (1.3129, 1.189) -> (3.0129, 1.189)
  line L7587 (0.2505, 0.4791) -> (0.4998, 0.8522)
  line L7588 (3.453, 1.1015) -> (3.8261, 0.8522)
  line L7589 (0.2505, -0.4011) -> (0.1629, 0.039)
  line L7590 (1.3129, -1.111) -> (0.8729, -1.0235)
  line L7591 (3.0129, 1.189) -> (3.453, 1.1015)
  line L7592 (3.0129, -1.111) -> (1.3129, -1.111)
  line L7593 (3.8261, -0.7742) -> (3.453, -1.0235)
  line L7594 (0.4998, -0.7742) -> (0.2505, -0.4011)
  line L7595 (1.3129, 1.189) -> (3.0129, 1.189)
  line L7596 (3.453, -1.0235) -> (3.0129, -1.111)
  line L7597 (1.3129, -1.111) -> (0.8729, -1.0235)
  line L7598 (4.0754, 0.4791) -> (4.1629, 0.039)
  line L7599 (0.2505, 0.4791) -> (0.4998, 0.8522)
  line L7600 (3.8261, 0.8522) -> (4.0754, 0.4791)
  line L7601 (0.1629, 0.039) -> (0.2505, 0.4791)
  line L7602 (0.2505, -0.4011) -> (0.1629, 0.039)
  line L7603 (0.8729, -1.0235) -> (0.4998, -0.7742)
  line L7604 (0.8729, 1.1015) -> (1.3129, 1.189)
  line L7605 (3.0129, 1.189) -> (3.453, 1.1015)
  line L7606 (3.8261, -0.7742) -> (3.453, -1.0235)
  line L7607 (3.0129, -1.111) -> (1.3129, -1.111)
  line L7608 (3.453, 1.1015) -> (3.8261, 0.8522)
  line L7609 (4.1629, 0.039) -> (4.0754, -0.4011)
  line L7610 (4.0754, -0.4011) -> (3.8261, -0.7742)
  line L7611 (0.4998, 0.8522) -> (0.8729, 1.1015)
  line L7612 (0.2505, 0.4791) -> (0.4998, 0.8522)
  line L7613 (0.2505, -0.4011) -> (0.1629, 0.039)
  line L7614 (3.0129, -1.111) -> (1.3129, -1.111)
  line L7615 (3.8261, -0.7742) -> (3.453, -1.0235)
  line L7616 (3.453, 1.1015) -> (3.8261, 0.8522)
  line L7617 (3.0129, 1.189) -> (3.453, 1.1015)
  line L7618 (0.8729, -1.0235) -> (0.4998, -0.7742)
  line L7619 (3.8261, 0.8522) -> (4.0754, 0.4791)
  line L7620 (1.3129, -1.111) -> (0.8729, -1.0235)
  line L7621 (3.453, -1.0235) -> (3.0129, -1.111)
  line L7622 (0.1629, 0.039) -> (0.2505, 0.4791)
  line L7623 (1.3129, 1.189) -> (3.0129, 1.189)
  line L7624 (0.4998, -0.7742) -> (0.2505, -0.4011)
  line L7625 (0.4998, 0.8522) -> (0.8729, 1.1015)
  line L7626 (4.1629, 0.039) -> (4.0754, -0.4011)
  line L7627 (4.0754, -0.4011) -> (3.8261, -0.7742)
  line L7628 (4.0754, 0.4791) -> (4.1629, 0.039)
  line L7629 (0.8729, 1.1015) -> (1.3129, 1.189)
  line L7630 (3.453, -12.0235) -> (3.0129, -12.111)
  line L7631 (1.3129, -12.111) -> (0.8729, -12.0235)
  line L7632 (4.0754, -11.4011) -> (3.8261, -11.7742)
  line L7633 (3.0129, -12.111) -> (1.3129, -12.111)
  line L7634 (0.2505, -10.5209) -> (0.4998, -10.1478)
  line L7635 (1.3129, -9.811) -> (3.0129, -9.811)
  line L7636 (4.0754, -10.5209) -> (4.1629, -10.961)
  line L7637 (0.2505, -11.4011) -> (0.1629, -10.961)
  line L7638 (4.1629, -10.961) -> (4.0754, -11.4011)
  line L7639 (3.8261, -11.7742) -> (3.453, -12.0235)
  line L7640 (0.4998, -10.1478) -> (0.8729, -9.8985)
  line L7641 (0.1629, -10.961) -> (0.2505, -10.5209)
  line L7642 (3.0129, -9.811) -> (3.453, -9.8985)
  line L7643 (3.453, -9.8985) -> (3.8261, -10.1478)
  line L7644 (0.4998, -11.7742) -> (0.2505, -11.4011)
  line L7645 (0.8729, -9.8985) -> (1.3129, -9.811)
  line L7646 (3.8261, -10.1478) -> (4.0754, -10.5209)
  line L7647 (0.8729, -12.0235) -> (0.4998, -11.7742)
  line L7648 (3.0129, -9.811) -> (3.453, -9.8985)
  line L7649 (0.2505, -11.4011) -> (0.1629, -10.961)
  line L7650 (3.8261, -10.1478) -> (4.0754, -10.5209)
  line L7651 (3.8261, -11.7742) -> (3.453, -12.0235)
  line L7652 (1.3129, -9.811) -> (3.0129, -9.811)
  line L7653 (3.453, -9.8985) -> (3.8261, -10.1478)
  line L7654 (3.0129, -12.111) -> (1.3129, -12.111)
  line L7655 (0.8729, -9.8985) -> (1.3129, -9.811)
  line L7656 (0.4998, -10.1478) -> (0.8729, -9.8985)
  line L7657 (0.1629, -10.961) -> (0.2505, -10.5209)
  line L7658 (4.1629, -10.961) -> (4.0754, -11.4011)
  line L7659 (0.2505, -10.5209) -> (0.4998, -10.1478)
  line L7660 (0.8729, -12.0235) -> (0.4998, -11.7742)
  line L7661 (3.453, -12.0235) -> (3.0129, -12.111)
  line L7662 (1.3129, -12.111) -> (0.8729, -12.0235)
  line L7663 (4.0754, -11.4011) -> (3.8261, -11.7742)
  line L7664 (0.4998, -11.7742) -> (0.2505, -11.4011)
  line L7665 (4.0754, -10.5209) -> (4.1629, -10.961)
  line L7666 (4.0754, -11.4011) -> (3.8261, -11.7742)
  line L7667 (3.0129, -12.111) -> (1.3129, -12.111)
  line L7668 (0.4998, -10.1478) -> (0.8729, -9.8985)
  line L7669 (0.2505, -10.5209) -> (0.4998, -10.1478)
  line L7670 (0.2505, -11.4011) -> (0.1629, -10.961)
  line L7671 (1.3129, -12.111) -> (0.8729, -12.0235)
  line L7672 (3.453, -12.0235) -> (3.0129, -12.111)
  line L7673 (0.8729, -9.8985) -> (1.3129, -9.811)
  line L7674 (3.453, -9.8985) -> (3.8261, -10.1478)
  line L7675 (4.0754, -10.5209) -> (4.1629, -10.961)
  line L7676 (0.8729, -12.0235) -> (0.4998, -11.7742)
  line L7677 (1.3129, -9.811) -> (3.0129, -9.811)
  line L7678 (4.1629, -10.961) -> (4.0754, -11.4011)
  line L7679 (0.1629, -10.961) -> (0.2505, -10.5209)
  line L7680 (3.8261, -11.7742) -> (3.453, -12.0235)
  line L7681 (3.8261, -10.1478) -> (4.0754, -10.5209)
  line L7682 (0.4998, -11.7742) -> (0.2505, -11.4011)
  line L7683 (3.0129, -9.811) -> (3.453, -9.8985)
  arc A1202 (195.9974, -61.2644) -> (194.7974, -61.2644) centre (195.3974, -61.2644) ccw
  arc A1203 (194.7974, -61.2644) -> (195.9974, -61.2644) centre (195.3974, -61.2644) ccw
  arc A1204 (194.7974, -61.2644) -> (195.9974, -61.2644) centre (195.3974, -61.2644) ccw
  arc A1205 (195.9974, -61.2644) -> (194.7974, -61.2644) centre (195.3974, -61.2644) ccw
  arc A1206 (194.7974, -61.2644) -> (195.9974, -61.2644) centre (195.3974, -61.2644) ccw
  arc A1207 (195.9974, -61.2644) -> (194.7974, -61.2644) centre (195.3974, -61.2644) ccw
  arc A1208 (192.4974, -63.5184) -> (191.2974, -63.5184) centre (191.8974, -63.5184) ccw
  arc A1209 (191.2974, -63.5184) -> (192.4974, -63.5184) centre (191.8974, -63.5184) ccw
  arc A1210 (191.2974, -63.5184) -> (192.4974, -63.5184) centre (191.8974, -63.5184) ccw
  arc A1211 (192.4974, -63.5184) -> (191.2974, -63.5184) centre (191.8974, -63.5184) ccw
  arc A1212 (191.2974, -63.5184) -> (192.4974, -63.5184) centre (191.8974, -63.5184) ccw
  arc A1213 (192.4974, -63.5184) -> (191.2974, -63.5184) centre (191.8974, -63.5184) ccw
  arc A1214 (175.7474, -80.3272) -> (176.9474, -80.3272) centre (176.3474, -80.3272) ccw
  arc A1215 (176.9474, -80.3272) -> (175.7474, -80.3272) centre (176.3474, -80.3272) ccw
  arc A1216 (175.7474, -80.3272) -> (176.9474, -80.3272) centre (176.3474, -80.3272) ccw
  arc A1217 (176.9474, -80.3272) -> (175.7474, -80.3272) centre (176.3474, -80.3272) ccw
  arc A1218 (175.7474, -80.3272) -> (176.9474, -80.3272) centre (176.3474, -80.3272) ccw
  arc A1219 (176.9474, -80.3272) -> (175.7474, -80.3272) centre (176.3474, -80.3272) ccw
  arc A1220 (172.2473, -82.5812) -> (173.4473, -82.5812) centre (172.8473, -82.5812) ccw
  arc A1221 (173.4473, -82.5812) -> (172.2473, -82.5812) centre (172.8473, -82.5812) ccw
  arc A1222 (172.2473, -82.5812) -> (173.4473, -82.5812) centre (172.8473, -82.5812) ccw
  arc A1223 (173.4473, -82.5812) -> (172.2473, -82.5812) centre (172.8473, -82.5812) ccw
  arc A1224 (173.4473, -82.5812) -> (172.2473, -82.5812) centre (172.8473, -82.5812) ccw
  arc A1225 (172.2473, -82.5812) -> (173.4473, -82.5812) centre (172.8473, -82.5812) ccw
  arc A1226 (176.9474, -61.2644) -> (175.7474, -61.2644) centre (176.3474, -61.2644) ccw
  arc A1227 (175.7474, -61.2644) -> (176.9474, -61.2644) centre (176.3474, -61.2644) ccw
  arc A1228 (176.9474, -61.2644) -> (175.7474, -61.2644) centre (176.3474, -61.2644) ccw
  arc A1229 (175.7474, -61.2644) -> (176.9474, -61.2644) centre (176.3474, -61.2644) ccw
  arc A1230 (176.9474, -61.2644) -> (175.7474, -61.2644) centre (176.3474, -61.2644) ccw
  arc A1231 (175.7474, -61.2644) -> (176.9474, -61.2644) centre (176.3474, -61.2644) ccw
  arc A1232 (173.4473, -63.5184) -> (172.2473, -63.5184) centre (172.8473, -63.5184) ccw
  arc A1233 (172.2473, -63.5184) -> (173.4473, -63.5184) centre (172.8473, -63.5184) ccw
  arc A1234 (173.4473, -63.5184) -> (172.2473, -63.5184) centre (172.8473, -63.5184) ccw
  arc A1235 (172.2473, -63.5184) -> (173.4473, -63.5184) centre (172.8473, -63.5184) ccw
  arc A1236 (172.2473, -63.5184) -> (173.4473, -63.5184) centre (172.8473, -63.5184) ccw
  arc A1237 (173.4473, -63.5184) -> (172.2473, -63.5184) centre (172.8473, -63.5184) ccw
  arc A1238 (175.7474, -42.2017) -> (176.9474, -42.2017) centre (176.3474, -42.2017) ccw
  arc A1239 (176.9474, -42.2017) -> (175.7474, -42.2017) centre (176.3474, -42.2017) ccw
  arc A1240 (175.7474, -42.2017) -> (176.9474, -42.2017) centre (176.3474, -42.2017) ccw
  arc A1241 (176.9474, -42.2017) -> (175.7474, -42.2017) centre (176.3474, -42.2017) ccw
  arc A1242 (176.9474, -42.2017) -> (175.7474, -42.2017) centre (176.3474, -42.2017) ccw
  arc A1243 (175.7474, -42.2017) -> (176.9474, -42.2017) centre (176.3474, -42.2017) ccw
  arc A1244 (173.4473, -44.4557) -> (172.2473, -44.4557) centre (172.8473, -44.4557) ccw
  arc A1245 (172.2473, -44.4557) -> (173.4473, -44.4557) centre (172.8473, -44.4557) ccw
  arc A1246 (172.2473, -44.4557) -> (173.4473, -44.4557) centre (172.8473, -44.4557) ccw
  arc A1247 (173.4473, -44.4557) -> (172.2473, -44.4557) centre (172.8473, -44.4557) ccw
  arc A1248 (172.2473, -44.4557) -> (173.4473, -44.4557) centre (172.8473, -44.4557) ccw
  arc A1249 (173.4473, -44.4557) -> (172.2473, -44.4557) centre (172.8473, -44.4557) ccw
  arc A1250 (176.9474, -23.1516) -> (175.7474, -23.1516) centre (176.3474, -23.1516) ccw
  arc A1251 (175.7474, -23.1516) -> (176.9474, -23.1516) centre (176.3474, -23.1516) ccw
  arc A1252 (176.9474, -23.1516) -> (175.7474, -23.1516) centre (176.3474, -23.1516) ccw
  arc A1253 (175.7474, -23.1516) -> (176.9474, -23.1516) centre (176.3474, -23.1516) ccw
  arc A1254 (176.9474, -23.1516) -> (175.7474, -23.1516) centre (176.3474, -23.1516) ccw
  arc A1255 (175.7474, -23.1516) -> (176.9474, -23.1516) centre (176.3474, -23.1516) ccw
  arc A1256 (173.4473, -25.4057) -> (172.2473, -25.4057) centre (172.8473, -25.4057) ccw
  arc A1257 (172.2473, -25.4057) -> (173.4473, -25.4057) centre (172.8473, -25.4057) ccw
  arc A1258 (173.4473, -25.4057) -> (172.2473, -25.4057) centre (172.8473, -25.4057) ccw
  arc A1259 (172.2473, -25.4057) -> (173.4473, -25.4057) centre (172.8473, -25.4057) ccw
  arc A1260 (172.2473, -25.4057) -> (173.4473, -25.4057) centre (172.8473, -25.4057) ccw
  arc A1261 (173.4473, -25.4057) -> (172.2473, -25.4057) centre (172.8473, -25.4057) ccw
  arc A1262 (156.6973, -80.3272) -> (157.8973, -80.3272) centre (157.2973, -80.3272) ccw
  arc A1263 (157.8973, -80.3272) -> (156.6973, -80.3272) centre (157.2973, -80.3272) ccw
  arc A1264 (156.6973, -80.3272) -> (157.8973, -80.3272) centre (157.2973, -80.3272) ccw
  arc A1265 (157.8973, -80.3272) -> (156.6973, -80.3272) centre (157.2973, -80.3272) ccw
  arc A1266 (156.6973, -80.3272) -> (157.8973, -80.3272) centre (157.2973, -80.3272) ccw
  arc A1267 (157.8973, -80.3272) -> (156.6973, -80.3272) centre (157.2973, -80.3272) ccw
  arc A1268 (154.3973, -82.5812) -> (153.1973, -82.5812) centre (153.7973, -82.5812) ccw
  arc A1269 (153.1973, -82.5812) -> (154.3973, -82.5812) centre (153.7973, -82.5812) ccw
  arc A1270 (153.1973, -82.5812) -> (154.3973, -82.5812) centre (153.7973, -82.5812) ccw
  arc A1271 (154.3973, -82.5812) -> (153.1973, -82.5812) centre (153.7973, -82.5812) ccw
  arc A1272 (153.1973, -82.5812) -> (154.3973, -82.5812) centre (153.7973, -82.5812) ccw
  arc A1273 (154.3973, -82.5812) -> (153.1973, -82.5812) centre (153.7973, -82.5812) ccw
  arc A1274 (156.6973, -42.2017) -> (157.8973, -42.2017) centre (157.2973, -42.2017) ccw
  arc A1275 (157.8973, -42.2017) -> (156.6973, -42.2017) centre (157.2973, -42.2017) ccw
  arc A1276 (157.8973, -42.2017) -> (156.6973, -42.2017) centre (157.2973, -42.2017) ccw
  arc A1277 (156.6973, -42.2017) -> (157.8973, -42.2017) centre (157.2973, -42.2017) ccw
  arc A1278 (156.6973, -42.2017) -> (157.8973, -42.2017) centre (157.2973, -42.2017) ccw
  arc A1279 (157.8973, -42.2017) -> (156.6973, -42.2017) centre (157.2973, -42.2017) ccw
  arc A1280 (154.3973, -44.4557) -> (153.1973, -44.4557) centre (153.7973, -44.4557) ccw
  arc A1281 (153.1973, -44.4557) -> (154.3973, -44.4557) centre (153.7973, -44.4557) ccw
  arc A1282 (154.3973, -44.4557) -> (153.1973, -44.4557) centre (153.7973, -44.4557) ccw
  arc A1283 (153.1973, -44.4557) -> (154.3973, -44.4557) centre (153.7973, -44.4557) ccw
  arc A1284 (154.3973, -44.4557) -> (153.1973, -44.4557) centre (153.7973, -44.4557) ccw
  arc A1285 (153.1973, -44.4557) -> (154.3973, -44.4557) centre (153.7973, -44.4557) ccw
  arc A1286 (157.8973, -61.2644) -> (156.6973, -61.2644) centre (157.2973, -61.2644) ccw
  arc A1287 (156.6973, -61.2644) -> (157.8973, -61.2644) centre (157.2973, -61.2644) ccw
  arc A1288 (156.6973, -61.2644) -> (157.8973, -61.2644) centre (157.2973, -61.2644) ccw
  arc A1289 (157.8973, -61.2644) -> (156.6973, -61.2644) centre (157.2973, -61.2644) ccw
  arc A1290 (156.6973, -61.2644) -> (157.8973, -61.2644) centre (157.2973, -61.2644) ccw
  arc A1291 (157.8973, -61.2644) -> (156.6973, -61.2644) centre (157.2973, -61.2644) ccw
  arc A1292 (154.3973, -63.5184) -> (153.1973, -63.5184) centre (153.7973, -63.5184) ccw
  arc A1293 (153.1973, -63.5184) -> (154.3973, -63.5184) centre (153.7973, -63.5184) ccw
  arc A1294 (154.3973, -63.5184) -> (153.1973, -63.5184) centre (153.7973, -63.5184) ccw
  arc A1295 (153.1973, -63.5184) -> (154.3973, -63.5184) centre (153.7973, -63.5184) ccw
  arc A1296 (154.3973, -63.5184) -> (153.1973, -63.5184) centre (153.7973, -63.5184) ccw
  arc A1297 (153.1973, -63.5184) -> (154.3973, -63.5184) centre (153.7973, -63.5184) ccw
  arc A1298 (157.8973, -23.1516) -> (156.6973, -23.1516) centre (157.2973, -23.1516) ccw
  arc A1299 (156.6973, -23.1516) -> (157.8973, -23.1516) centre (157.2973, -23.1516) ccw
  arc A1300 (156.6973, -23.1516) -> (157.8973, -23.1516) centre (157.2973, -23.1516) ccw
  arc A1301 (157.8973, -23.1516) -> (156.6973, -23.1516) centre (157.2973, -23.1516) ccw
  arc A1302 (156.6973, -23.1516) -> (157.8973, -23.1516) centre (157.2973, -23.1516) ccw
  arc A1303 (157.8973, -23.1516) -> (156.6973, -23.1516) centre (157.2973, -23.1516) ccw
  arc A1304 (154.3973, -25.4057) -> (153.1973, -25.4057) centre (153.7973, -25.4057) ccw
  arc A1305 (153.1973, -25.4057) -> (154.3973, -25.4057) centre (153.7973, -25.4057) ccw
  arc A1306 (153.1973, -25.4057) -> (154.3973, -25.4057) centre (153.7973, -25.4057) ccw
  arc A1307 (154.3973, -25.4057) -> (153.1973, -25.4057) centre (153.7973, -25.4057) ccw
  arc A1308 (154.3973, -25.4057) -> (153.1973, -25.4057) centre (153.7973, -25.4057) ccw
  arc A1309 (153.1973, -25.4057) -> (154.3973, -25.4057) centre (153.7973, -25.4057) ccw
  arc A1310 (137.6473, -61.2644) -> (138.8473, -61.2644) centre (138.2473, -61.2644) ccw
  arc A1311 (138.8473, -61.2644) -> (137.6473, -61.2644) centre (138.2473, -61.2644) ccw
  arc A1312 (138.8473, -61.2644) -> (137.6473, -61.2644) centre (138.2473, -61.2644) ccw
  arc A1313 (137.6473, -61.2644) -> (138.8473, -61.2644) centre (138.2473, -61.2644) ccw
  arc A1314 (138.8473, -61.2644) -> (137.6473, -61.2644) centre (138.2473, -61.2644) ccw
  arc A1315 (137.6473, -61.2644) -> (138.8473, -61.2644) centre (138.2473, -61.2644) ccw
  arc A1316 (134.1473, -63.5184) -> (135.3473, -63.5184) centre (134.7473, -63.5184) ccw
  arc A1317 (135.3473, -63.5184) -> (134.1473, -63.5184) centre (134.7473, -63.5184) ccw
  arc A1318 (135.3473, -63.5184) -> (134.1473, -63.5184) centre (134.7473, -63.5184) ccw
  arc A1319 (134.1473, -63.5184) -> (135.3473, -63.5184) centre (134.7473, -63.5184) ccw
  arc A1320 (134.1473, -63.5184) -> (135.3473, -63.5184) centre (134.7473, -63.5184) ccw
  arc A1321 (135.3473, -63.5184) -> (134.1473, -63.5184) centre (134.7473, -63.5184) ccw
  arc A1322 (138.8473, -42.2017) -> (137.6473, -42.2017) centre (138.2473, -42.2017) ccw
  arc A1323 (137.6473, -42.2017) -> (138.8473, -42.2017) centre (138.2473, -42.2017) ccw
  arc A1324 (138.8473, -42.2017) -> (137.6473, -42.2017) centre (138.2473, -42.2017) ccw
  arc A1325 (137.6473, -42.2017) -> (138.8473, -42.2017) centre (138.2473, -42.2017) ccw
  arc A1326 (137.6473, -42.2017) -> (138.8473, -42.2017) centre (138.2473, -42.2017) ccw
  arc A1327 (138.8473, -42.2017) -> (137.6473, -42.2017) centre (138.2473, -42.2017) ccw
  arc A1328 (135.3473, -44.4557) -> (134.1473, -44.4557) centre (134.7473, -44.4557) ccw
  arc A1329 (134.1473, -44.4557) -> (135.3473, -44.4557) centre (134.7473, -44.4557) ccw
  arc A1330 (134.1473, -44.4557) -> (135.3473, -44.4557) centre (134.7473, -44.4557) ccw
  arc A1331 (135.3473, -44.4557) -> (134.1473, -44.4557) centre (134.7473, -44.4557) ccw
  arc A1332 (134.1473, -44.4557) -> (135.3473, -44.4557) centre (134.7473, -44.4557) ccw
  arc A1333 (135.3473, -44.4557) -> (134.1473, -44.4557) centre (134.7473, -44.4557) ccw
  arc A1334 (138.8473, -23.1516) -> (137.6473, -23.1516) centre (138.2473, -23.1516) ccw
  arc A1335 (137.6473, -23.1516) -> (138.8473, -23.1516) centre (138.2473, -23.1516) ccw
  arc A1336 (138.8473, -23.1516) -> (137.6473, -23.1516) centre (138.2473, -23.1516) ccw
  arc A1337 (137.6473, -23.1516) -> (138.8473, -23.1516) centre (138.2473, -23.1516) ccw
  arc A1338 (137.6473, -23.1516) -> (138.8473, -23.1516) centre (138.2473, -23.1516) ccw
  arc A1339 (138.8473, -23.1516) -> (137.6473, -23.1516) centre (138.2473, -23.1516) ccw
  arc A1340 (134.1473, -25.4057) -> (135.3473, -25.4057) centre (134.7473, -25.4057) ccw
  arc A1341 (135.3473, -25.4057) -> (134.1473, -25.4057) centre (134.7473, -25.4057) ccw
  arc A1342 (135.3473, -25.4057) -> (134.1473, -25.4057) centre (134.7473, -25.4057) ccw
  arc A1343 (134.1473, -25.4057) -> (135.3473, -25.4057) centre (134.7473, -25.4057) ccw
  arc A1344 (134.1473, -25.4057) -> (135.3473, -25.4057) centre (134.7473, -25.4057) ccw
  arc A1345 (135.3473, -25.4057) -> (134.1473, -25.4057) centre (134.7473, -25.4057) ccw
  arc A1346 (137.6473, -80.3272) -> (138.8473, -80.3272) centre (138.2473, -80.3272) ccw
  arc A1347 (138.8473, -80.3272) -> (137.6473, -80.3272) centre (138.2473, -80.3272) ccw
  arc A1348 (138.8473, -80.3272) -> (137.6473, -80.3272) centre (138.2473, -80.3272) ccw
  arc A1349 (137.6473, -80.3272) -> (138.8473, -80.3272) centre (138.2473, -80.3272) ccw
  arc A1350 (137.6473, -80.3272) -> (138.8473, -80.3272) centre (138.2473, -80.3272) ccw
  arc A1351 (138.8473, -80.3272) -> (137.6473, -80.3272) centre (138.2473, -80.3272) ccw
  arc A1352 (134.1473, -82.5812) -> (135.3473, -82.5812) centre (134.7473, -82.5812) ccw
  arc A1353 (135.3473, -82.5812) -> (134.1473, -82.5812) centre (134.7473, -82.5812) ccw
  arc A1354 (134.1473, -82.5812) -> (135.3473, -82.5812) centre (134.7473, -82.5812) ccw
  arc A1355 (135.3473, -82.5812) -> (134.1473, -82.5812) centre (134.7473, -82.5812) ccw
  arc A1356 (135.3473, -82.5812) -> (134.1473, -82.5812) centre (134.7473, -82.5812) ccw
  arc A1357 (134.1473, -82.5812) -> (135.3473, -82.5812) centre (134.7473, -82.5812) ccw
  arc A1358 (118.5972, -80.3272) -> (119.7972, -80.3272) centre (119.1972, -80.3272) ccw
  arc A1359 (119.7972, -80.3272) -> (118.5972, -80.3272) centre (119.1972, -80.3272) ccw
  arc A1360 (118.5972, -80.3272) -> (119.7972, -80.3272) centre (119.1972, -80.3272) ccw
  arc A1361 (119.7972, -80.3272) -> (118.5972, -80.3272) centre (119.1972, -80.3272) ccw
  arc A1362 (118.5972, -80.3272) -> (119.7972, -80.3272) centre (119.1972, -80.3272) ccw
  arc A1363 (119.7972, -80.3272) -> (118.5972, -80.3272) centre (119.1972, -80.3272) ccw
  arc A1364 (115.0972, -82.5812) -> (116.2972, -82.5812) centre (115.6972, -82.5812) ccw
  arc A1365 (116.2972, -82.5812) -> (115.0972, -82.5812) centre (115.6972, -82.5812) ccw
  arc A1366 (116.2972, -82.5812) -> (115.0972, -82.5812) centre (115.6972, -82.5812) ccw
  arc A1367 (115.0972, -82.5812) -> (116.2972, -82.5812) centre (115.6972, -82.5812) ccw
  arc A1368 (116.2972, -82.5812) -> (115.0972, -82.5812) centre (115.6972, -82.5812) ccw
  arc A1369 (115.0972, -82.5812) -> (116.2972, -82.5812) centre (115.6972, -82.5812) ccw
  arc A1370 (119.7972, -61.2644) -> (118.5972, -61.2644) centre (119.1972, -61.2644) ccw
  arc A1371 (118.5972, -61.2644) -> (119.7972, -61.2644) centre (119.1972, -61.2644) ccw
  arc A1372 (119.7972, -61.2644) -> (118.5972, -61.2644) centre (119.1972, -61.2644) ccw
  arc A1373 (118.5972, -61.2644) -> (119.7972, -61.2644) centre (119.1972, -61.2644) ccw
  arc A1374 (119.7972, -61.2644) -> (118.5972, -61.2644) centre (119.1972, -61.2644) ccw
  arc A1375 (118.5972, -61.2644) -> (119.7972, -61.2644) centre (119.1972, -61.2644) ccw
  arc A1376 (116.2972, -63.5184) -> (115.0972, -63.5184) centre (115.6972, -63.5184) ccw
  arc A1377 (115.0972, -63.5184) -> (116.2972, -63.5184) centre (115.6972, -63.5184) ccw
  arc A1378 (116.2972, -63.5184) -> (115.0972, -63.5184) centre (115.6972, -63.5184) ccw
  arc A1379 (115.0972, -63.5184) -> (116.2972, -63.5184) centre (115.6972, -63.5184) ccw
  arc A1380 (116.2972, -63.5184) -> (115.0972, -63.5184) centre (115.6972, -63.5184) ccw
  arc A1381 (115.0972, -63.5184) -> (116.2972, -63.5184) centre (115.6972, -63.5184) ccw
  arc A1382 (119.7972, -23.1516) -> (118.5972, -23.1516) centre (119.1972, -23.1516) ccw
  arc A1383 (118.5972, -23.1516) -> (119.7972, -23.1516) centre (119.1972, -23.1516) ccw
  arc A1384 (119.7972, -23.1516) -> (118.5972, -23.1516) centre (119.1972, -23.1516) ccw
  arc A1385 (118.5972, -23.1516) -> (119.7972, -23.1516) centre (119.1972, -23.1516) ccw
  arc A1386 (119.7972, -23.1516) -> (118.5972, -23.1516) centre (119.1972, -23.1516) ccw
  arc A1387 (118.5972, -23.1516) -> (119.7972, -23.1516) centre (119.1972, -23.1516) ccw
  arc A1388 (116.2972, -25.4057) -> (115.0972, -25.4057) centre (115.6972, -25.4057) ccw
  arc A1389 (115.0972, -25.4057) -> (116.2972, -25.4057) centre (115.6972, -25.4057) ccw
  arc A1390 (116.2972, -25.4057) -> (115.0972, -25.4057) centre (115.6972, -25.4057) ccw
  arc A1391 (115.0972, -25.4057) -> (116.2972, -25.4057) centre (115.6972, -25.4057) ccw
  arc A1392 (115.0972, -25.4057) -> (116.2972, -25.4057) centre (115.6972, -25.4057) ccw
  arc A1393 (116.2972, -25.4057) -> (115.0972, -25.4057) centre (115.6972, -25.4057) ccw
  arc A1394 (118.5972, -42.2017) -> (119.7972, -42.2017) centre (119.1972, -42.2017) ccw